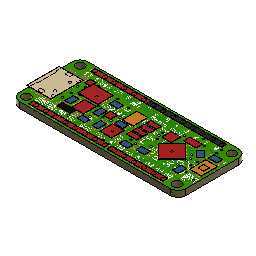
PortableEnclosure (Autodesk Fusion 360 archive; units mm, degrees)
design "Metro Mini Rev B"
part number: 20609
part number: 0.1uF
part number: YELLOW
part number: FIDUCIAL""
part number: CSTCE16M0V53-R0 16MHZ
part number: KMR2
part number: 20610
part number: MBR120
part number: 1K
part number: MIC5225-3.3
part number: ATMEGA328P
part number: CP2104
part number: 20329
Autodesk Fusion 360 part; units mm, degrees
sketch "sketch 301" plane through (0, 0, 0) normal (0, 0, 1) x (1, 0, 0)
  line L0 (0, 15.748) -> (0, 11.684)
  line L1 (0, 11.684) -> (0.254, 11.43)
  line L2 (0.254, 11.43) -> (0.254, 6.604)
  line L3 (0.254, 6.604) -> (0, 6.35)
  line L4 (0, 6.35) -> (0, 2.032)
  arc A0 (0, 2.032) -> (2.032, 0) centre (2.032, 2.032) ccw
  line L5 (2.032, 0) -> (41.148, 0)
  arc A1 (41.148, 0) -> (43.18, 2.032) centre (41.148, 2.032) ccw
  line L6 (43.18, 2.032) -> (43.18, 15.748)
  arc A2 (43.18, 15.748) -> (41.148, 17.78) centre (41.148, 15.748) ccw
  line L7 (41.148, 17.78) -> (2.032, 17.78)
  arc A3 (2.032, 17.78) -> (0, 15.748) centre (2.032, 15.748) ccw
  circle A4 centre (1.905, 15.875) radius 1.1
  circle A5 centre (1.905, 1.905) radius 1.1
  circle A6 centre (41.275, 15.875) radius 1.1
  circle A7 centre (41.021, 1.905) radius 1.1
  arc A8 (3.068, 12.59) -> (2.718, 12.94) centre (2.718, 12.59) ccw
  line L8 (3.068, 12.59) -> (3.068, 12.39)
  arc A9 (2.718, 12.04) -> (3.068, 12.39) centre (2.718, 12.39) ccw
  line L9 (2.718, 12.04) -> (2.168, 12.04)
  arc A10 (1.768, 12.39) -> (2.168, 12.04) centre (2.143, 12.415) ccw
  line L10 (1.768, 12.39) -> (1.768, 12.59)
  arc A11 (2.168, 12.94) -> (1.768, 12.59) centre (2.143, 12.565) ccw
  line L11 (2.168, 12.94) -> (2.718, 12.94)
  arc A12 (2.718, 4.84) -> (3.068, 5.29) centre (2.668, 5.24) ccw
  line L12 (2.718, 4.84) -> (2.118, 4.84)
  arc A13 (1.768, 5.29) -> (2.118, 4.84) centre (2.168, 5.24) ccw
  arc A14 (2.118, 5.74) -> (1.768, 5.29) centre (2.168, 5.34) ccw
  line L13 (2.118, 5.74) -> (2.718, 5.74)
  arc A15 (3.068, 5.29) -> (2.718, 5.74) centre (2.668, 5.34) ccw
extrude "Board" add sketch "sketch 301" along normal blind 1.57 makes body 1 in component "Board"
sketch "sketch 1110" plane through (0, 0, 0) normal (0, 0, 1) x (1, 0, 0)
  line L0 (-7.62, -0.635) -> (6.85, -0.635)
  line L1 (6.85, -0.635) -> (6.85, 0.635)
  line L2 (6.85, 0.635) -> (-7.62, 0.635)
  line L3 (-7.62, 0.635) -> (-7.62, -0.635)
extrude "1X06_ROUND" add sketch "sketch 1110" along normal blind 0.1 separate body makes body 2 in component "1X06_ROUND"
sketch "sketch 1313" plane through (0, 0, 0) normal (0, 0, 1) x (1, 0, 0)
  line L0 (-1.092, -0.724) -> (1.106, -0.724)
  line L1 (1.106, -0.724) -> (1.106, 0.726)
  line L2 (1.106, 0.726) -> (-1.092, 0.726)
  line L3 (-1.092, 0.726) -> (-1.092, -0.724)
extrude "0805-NO" add sketch "sketch 1313" along normal blind 0.1 separate body makes body 3 in component "0805-NO"
sketch "sketch 1468" plane through (0, 0, 0) normal (0, 0, 1) x (1, 0, 0)
  line L0 (-0.625, -1.3334) -> (0.625, -1.3334)
  line L1 (0.625, -1.3334) -> (0.625, 1.3334)
  line L2 (0.625, 1.3334) -> (-0.625, 1.3334)
  line L3 (-0.625, 1.3334) -> (-0.625, -1.3334)
extrude "CHIPLED_0805_NOOUTLINE" add sketch "sketch 1468" along normal blind 0.1 separate body makes body 4 in component "CHIPLED_0805_NOOUTLINE"
sketch "sketch 1607" plane through (0, 0, 0) normal (0, 0, 1) x (1, 0, 0)
  line L0 (-0.75, -0.75) -> (0.75, -0.75)
  line L1 (0.75, -0.75) -> (0.75, 0.75)
  line L2 (0.75, 0.75) -> (-0.75, 0.75)
  line L3 (-0.75, 0.75) -> (-0.75, -0.75)
extrude "FIDUCIAL_1MM" add sketch "sketch 1607" along normal blind 0.1 separate body makes body 5 in component "FIDUCIAL_1MM"
sketch "sketch 1738" plane through (0, 0, 0) normal (0, 0, 1) x (1, 0, 0)
  line L0 (-1, -0.65) -> (1, -0.65)
  line L1 (1, -0.65) -> (1, 0.65)
  line L2 (1, 0.65) -> (-1, 0.65)
  line L3 (-1, 0.65) -> (-1, -0.65)
extrude "_0805MP" add sketch "sketch 1738" along normal blind 0.1 separate body makes body 6 in component "_0805MP"
sketch "sketch 1869" plane through (0, 0, 0) normal (0, 0, 1) x (1, 0, 0)
  line L0 (-1.6, -0.8) -> (1.6, -0.8)
  line L1 (1.6, -0.8) -> (1.6, 0.8)
  line L2 (1.6, 0.8) -> (-1.6, 0.8)
  line L3 (-1.6, 0.8) -> (-1.6, -0.8)
extrude "RESONATOR" add sketch "sketch 1869" along normal blind 0.1 separate body makes body 7 in component "RESONATOR"
sketch "sketch 2000" plane through (0, 0, 0) normal (0, 0, 1) x (1, 0, 0)
  line L0 (-2.1, -1.525) -> (2.1, -1.525)
  line L1 (2.1, -1.525) -> (2.1, 1.525)
  line L2 (2.1, 1.525) -> (-2.1, 1.525)
  line L3 (-2.1, 1.525) -> (-2.1, -1.525)
extrude "BTN_KMR2_4.6X2.8" add sketch "sketch 2000" along normal blind 0.1 separate body makes body 8 in component "BTN_KMR2_4.6X2.8"
sketch "sketch 2131" plane through (0, 0, 0) normal (0, 0, 1) x (1, 0, 0)
  line L0 (-10.16, -0.635) -> (9.39, -0.635)
  line L1 (9.39, -0.635) -> (9.39, 0.635)
  line L2 (9.39, 0.635) -> (-10.16, 0.635)
  line L3 (-10.16, 0.635) -> (-10.16, -0.635)
extrude "1X08_ROUND" add sketch "sketch 2131" along normal blind 0.1 separate body makes body 9 in component "1X08_ROUND"
sketch "sketch 2262" plane through (0, 0, 0) normal (0, 0, 1) x (1, 0, 0)
  line L0 (-2.286, -1.016) -> (2.286, -1.016)
  line L1 (2.286, -1.016) -> (2.286, 1.016)
  line L2 (2.286, 1.016) -> (-2.286, 1.016)
  line L3 (-2.286, 1.016) -> (-2.286, -1.016)
extrude "SOLDERJUMPER_2WAY_OPEN_NOPASTE" add sketch "sketch 2262" along normal blind 0.1 separate body makes body 10 in component "SOLDERJUMPER_2WAY_OPEN_NOPASTE"
sketch "sketch 2393" plane through (0, 0, 0) normal (0, 0, 1) x (1, 0, 0)
  line L0 (-1.723, -0.7) -> (1.723, -0.7)
  line L1 (1.723, -0.7) -> (1.723, 0.7)
  line L2 (1.723, 0.7) -> (-1.723, 0.7)
  line L3 (-1.723, 0.7) -> (-1.723, -0.7)
extrude "SOD-123" add sketch "sketch 2393" along normal blind 0.1 separate body makes body 11 in component "SOD-123"
sketch "sketch 2524" plane through (0, 0, 0) normal (0, 0, 1) x (1, 0, 0)
  line L0 (-1.9, -1.4) -> (1.9, -1.4)
  line L1 (1.9, -1.4) -> (1.9, 1.4)
  line L2 (1.9, 1.4) -> (-1.9, 1.4)
  line L3 (-1.9, 1.4) -> (-1.9, -1.4)
extrude "RESPACK_4X0603" add sketch "sketch 2524" along normal blind 0.1 separate body makes body 12 in component "RESPACK_4X0603"
sketch "sketch 2663" plane through (0, 0, 0) normal (0, 0, 1) x (1, 0, 0)
  line L0 (-1.65, -1.5) -> (1.65, -1.5)
  line L1 (1.65, -1.5) -> (1.65, 1.5)
  line L2 (1.65, 1.5) -> (-1.65, 1.5)
  line L3 (-1.65, 1.5) -> (-1.65, -1.5)
extrude "SOT23-5" add sketch "sketch 2663" along normal blind 0.1 separate body makes body 13 in component "SOT23-5"
sketch "sketch 2794" plane through (0, 0, 0) normal (0, 0, 1) x (1, 0, 0)
  line L0 (-2.5, -2.5) -> (2.5, -2.5)
  line L1 (2.5, -2.5) -> (2.5, 2.5)
  line L2 (2.5, 2.5) -> (-2.5, 2.5)
  line L3 (-2.5, 2.5) -> (-2.5, -2.5)
extrude "MLF32-TH" add sketch "sketch 2794" along normal blind 0.1 separate body makes body 14 in component "MLF32-TH"
sketch "sketch 2925" plane through (0, 0, 0) normal (0, 0, 1) x (1, 0, 0)
  line L0 (-10.16, -0.635) -> (9.39, -0.635)
  line L1 (9.39, -0.635) -> (9.39, 0.635)
  line L2 (9.39, 0.635) -> (-10.16, 0.635)
  line L3 (-10.16, 0.635) -> (-10.16, -0.635)
extrude "1X08_ROUND_70" add sketch "sketch 2925" along normal blind 0.1 separate body makes body 15 in component "1X08_ROUND_70"
sketch "sketch 3056" plane through (0, 0, 0) normal (0, 0, 1) x (1, 0, 0)
  line L0 (-0.002, -0.002) -> (2.436, -0.002)
  line L1 (2.436, -0.002) -> (2.436, 2.433)
  line L2 (2.436, 2.433) -> (-0.002, 2.433)
  line L3 (-0.002, 2.433) -> (-0.002, -0.002)
extrude "ADAFRUIT_2.5MM" add sketch "sketch 3056" along normal blind 0.1 separate body makes body 16 in component "ADAFRUIT_2.5MM"
sketch "sketch 3187" plane through (0, 0, 0) normal (0, 0, 1) x (1, 0, 0)
  line L0 (0.013, 0.013) -> (25.336, 0.013)
  line L1 (25.336, 0.013) -> (25.336, 12.764)
  line L2 (25.336, 12.764) -> (0.013, 12.764)
  line L3 (0.013, 12.764) -> (0.013, 0.013)
extrude "METROMINI_SILK" add sketch "sketch 3187" along normal blind 0.1 separate body makes body 17 in component "METROMINI_SILK"
sketch "sketch 3318" plane through (0, 0, 0) normal (0, 0, 1) x (1, 0, 0)
  line L0 (-0.004, -0.004) -> (4.873, -0.004)
  line L1 (4.873, -0.004) -> (4.873, 4.865)
  line L2 (4.873, 4.865) -> (-0.004, 4.865)
  line L3 (-0.004, 4.865) -> (-0.004, -0.004)
extrude "ADAFRUIT_5MM" add sketch "sketch 3318" along normal blind 0.1 separate body makes body 18 in component "ADAFRUIT_5MM"
sketch "sketch 3449" plane through (0, 0, 0) normal (0, 0, 1) x (1, 0, 0)
  line L0 (-0.006, -0.006) -> (4.032, -0.006)
  line L1 (4.032, -0.006) -> (4.032, 2.877)
  line L2 (4.032, 2.877) -> (-0.006, 2.877)
  line L3 (-0.006, 2.877) -> (-0.006, -0.006)
extrude "SYMBOL_CE_TINY" add sketch "sketch 3449" along normal blind 0.1 separate body makes body 19 in component "SYMBOL_CE_TINY"
sketch "sketch 3580" plane through (0, 0, 0) normal (0, 0, 1) x (1, 0, 0)
  line L0 (-0.006, -0.006) -> (3.981, -0.006)
  line L1 (3.981, -0.006) -> (3.981, 2.838)
  line L2 (3.981, 2.838) -> (-0.006, 2.838)
  line L3 (-0.006, 2.838) -> (-0.006, -0.006)
extrude "SYMBOL_FCC_TINY" add sketch "sketch 3580" along normal blind 0.1 separate body makes body 20 in component "SYMBOL_FCC_TINY"
sketch "sketch 3711" plane through (0, 0, 0) normal (0, 0, 1) x (1, 0, 0)
  line L0 (-3.175, -2) -> (2, -2)
  line L1 (2, -2) -> (2, 2)
  line L2 (2, 2) -> (-3.175, 2)
  line L3 (-3.175, 2) -> (-3.175, -2)
extrude "QFN24_4MM_SMSC" add sketch "sketch 3711" along normal blind 0.1 separate body makes body 21 in component "QFN24_4MM_SMSC"
sketch "sketch 3842" plane through (0, 0, 0) normal (0, 0, 1) x (1, 0, 0)
  line L0 (-4.05, -4.9) -> (4.35, -4.9)
  line L1 (4.35, -4.9) -> (4.35, 1.3)
  line L2 (4.35, 1.3) -> (-4.05, 1.3)
  line L3 (-4.05, 1.3) -> (-4.05, -4.9)
extrude "4UCONN_20329_V2" add sketch "sketch 3842" along normal blind 0.1 separate body makes body 22 in component "4UCONN_20329_V2"
sketch "sketch 3973" plane through (0, 0, 0) normal (0, 0, 1) x (1, 0, 0)
  line L0 (-0.898, -0.898) -> (0.898, -0.898)
  line L1 (0.898, -0.898) -> (0.898, 0.898)
  line L2 (0.898, 0.898) -> (-0.898, 0.898)
  line L3 (-0.898, 0.898) -> (-0.898, -0.898)
extrude "PCBFEAT-REV-040" add sketch "sketch 3973" along normal blind 0.1 separate body makes body 23 in component "PCBFEAT-REV-040"
sketch "sketch 559" plane through (0, 0, 0) normal (0, 0, 1) x (1, 0, 0)
  circle A0 centre (25.146, 5.842) radius 0.2415
  circle A1 centre (14.605, 5.715) radius 0.2415
  circle A2 centre (33.02, 8.509) radius 0.25
  circle A3 centre (39.116, 15.24) radius 0.2415
  circle A4 centre (9.271, 4.318) radius 0.2415
  circle A5 centre (21.59, 2.286) radius 0.2415
  circle A6 centre (34.29, 15.367) radius 0.2415
  circle A7 centre (38.735, 9.525) radius 0.2415
  circle A8 centre (20.701, 5.461) radius 0.2415
  circle A9 centre (26.543, 5.588) radius 0.2415
  circle A10 centre (18.669, 9.398) radius 0.2415
  circle A11 centre (10.922, 11.176) radius 0.2415
  circle A12 centre (36.068, 13.97) radius 0.2415
  circle A13 centre (11.557, 3.175) radius 0.2415
  circle A14 centre (42.291, 4.826) radius 0.2415
  circle A15 centre (28.321, 9.398) radius 0.2415
  circle A16 centre (27.686, 11.557) radius 0.2415
  circle A17 centre (16.383, 7.239) radius 0.2415
  circle A18 centre (8.763, 13.716) radius 0.25
  circle A19 centre (36.957, 8.382) radius 0.197
  circle A20 centre (36.703, 6.35) radius 0.197
  circle A21 centre (37.084, 9.398) radius 0.197
  circle A22 centre (36.322, 10.414) radius 0.197
  circle A23 centre (31.115, 13.716) radius 0.2415
  circle A24 centre (8.382, 9.398) radius 0.25
  circle A25 centre (13.335, 9.271) radius 0.25
  circle A26 centre (39.497, 5.715) radius 0.197
  circle A27 centre (17.653, 12.7) radius 0.2415
  circle A28 centre (38.608, 7.874) radius 0.197
  circle A29 centre (14.224, 13.335) radius 0.2415
  circle A30 centre (6.223, 10.922) radius 0.2415
  circle A31 centre (6.731, 6.477) radius 0.2415
  circle A32 centre (29.21, 6.985) radius 0.2415
  circle A33 centre (18.161, 7.62) radius 0.2415
  circle A34 centre (39.243, 13.97) radius 0.2415
  circle A35 centre (27.813, 10.414) radius 0.2415
  circle A36 centre (6.858, 8.636) radius 0.25
  circle A37 centre (7.366, 11.811) radius 0.25
  circle A38 centre (25.4, 1.27) radius 0.5
  circle A39 centre (27.94, 1.27) radius 0.5
  circle A40 centre (30.48, 1.27) radius 0.5
  circle A41 centre (33.02, 1.27) radius 0.5
  circle A42 centre (35.56, 1.27) radius 0.5
  circle A43 centre (38.1, 1.27) radius 0.5
  circle A44 centre (17.78, 16.51) radius 0.5
  circle A45 centre (15.24, 16.51) radius 0.5
  circle A46 centre (12.7, 16.51) radius 0.5
  circle A47 centre (10.16, 16.51) radius 0.5
  circle A48 centre (7.62, 16.51) radius 0.5
  circle A49 centre (5.08, 16.51) radius 0.5
  circle A50 centre (20.32, 16.51) radius 0.5
  circle A51 centre (22.86, 16.51) radius 0.5
  circle A52 centre (25.4, 16.51) radius 0.5
  circle A53 centre (27.94, 16.51) radius 0.5
  circle A54 centre (30.48, 16.51) radius 0.5
  circle A55 centre (33.02, 16.51) radius 0.5
  circle A56 centre (35.56, 16.51) radius 0.5
  circle A57 centre (38.1, 16.51) radius 0.5
  circle A58 centre (5.08, 1.27) radius 0.5
  circle A59 centre (7.62, 1.27) radius 0.5
  circle A60 centre (10.16, 1.27) radius 0.5
  circle A61 centre (12.7, 1.27) radius 0.5
  circle A62 centre (15.24, 1.27) radius 0.5
  circle A63 centre (17.78, 1.27) radius 0.5
  circle A64 centre (20.32, 1.27) radius 0.5
  circle A65 centre (22.86, 1.27) radius 0.5
  circle A66 centre (4.318, 10.84) radius 0.35
  circle A67 centre (4.318, 6.94) radius 0.35
  circle A68 centre (2.418, 5.29) radius 0.45
  circle A69 centre (2.418, 12.49) radius 0.45
  circle A70 centre (5.218, 12.19) radius 0.4
  circle A71 centre (5.218, 5.59) radius 0.4
extrude "Extrude2" cut sketch "sketch 559" along normal blind 1.57 bodies 1 in component "Board"
component "PCB Component" placed x (1, 0, 0) y (0, 1, 0) z (0, 0, 1) at (0, 0, 0)
component "Board" placed x (1, 0, 0) y (0, 1, 0) z (0, 0, 1) at (0, 0, 0) in component "PCB Component"
component "1X06_ROUND" placed x (1, 0, 0) y (0, 1, 0) z (0, 0, 1) at (31.75, 1.27, 1.57) in component "PCB Component"
component "1X06_ROUND" placed x (-1, 0, 0) y (0, -1, 0) z (0, 0, 1) at (11.43, 16.51, 1.57) in component "PCB Component"
component "0805-NO" placed x (0, -1, 0) y (1, 0, 0) z (0, 0, 1) at (17.653, 5.08, 1.57) in component "PCB Component"
component "0805-NO" placed x (1, 0, 0) y (0, 1, 0) z (0, 0, 1) at (29.148, 4.931, 1.57) in component "PCB Component"
component "0805-NO" placed x (-1, 0, 0) y (0, -1, 0) z (0, 0, 1) at (20.447, 8.001, 1.57) in component "PCB Component"
component "0805-NO" placed x (0, 1, 0) y (-1, 0, 0) z (0, 0, 1) at (8.509, 7.112, 1.57) in component "PCB Component"
component "0805-NO" placed x (-0.707107, 0.707107, 0) y (-0.707107, -0.707107, 0) z (0, 0, 1) at (37.27, 11.603, 1.57) in component "PCB Component"
component "0805-NO" placed x (1, 0, 0) y (0, 1, 0) z (0, 0, 1) at (25.527, 4.191, 1.57) in component "PCB Component"
component "0805-NO" placed x (1, 0, 0) y (0, 1, 0) z (0, 0, 1) at (40.386, 12.446, 1.57) in component "PCB Component"
component "0805-NO" placed x (0, -1, 0) y (1, 0, 0) z (0, 0, 1) at (38.1, 5.461, 1.57) in component "PCB Component"
component "0805-NO" placed x (1, 0, 0) y (0, 1, 0) z (0, 0, 1) at (15.367, 11.811, 1.57) in component "PCB Component"
component "0805-NO" placed x (0, -1, 0) y (1, 0, 0) z (0, 0, 1) at (14.859, 8.001, 1.57) in component "PCB Component"
component "CHIPLED_0805_NOOUTLINE" placed x (0, 1, 0) y (-1, 0, 0) z (0, 0, 1) at (24.638, 8.763, 1.57) in component "PCB Component"
component "CHIPLED_0805_NOOUTLINE" placed x (0, 1, 0) y (-1, 0, 0) z (0, 0, 1) at (24.638, 7.112, 1.57) in component "PCB Component"
component "CHIPLED_0805_NOOUTLINE" placed x (0, 1, 0) y (-1, 0, 0) z (0, 0, 1) at (24.765, 10.414, 1.57) in component "PCB Component"
component "CHIPLED_0805_NOOUTLINE" placed x (0, 1, 0) y (-1, 0, 0) z (0, 0, 1) at (24.765, 12.065, 1.57) in component "PCB Component"
component "FIDUCIAL_1MM" placed x (1, 0, 0) y (0, 1, 0) z (0, 0, 1) at (7.112, 13.335, 1.57) in component "PCB Component"
component "FIDUCIAL_1MM" placed x (1, 0, 0) y (0, 1, 0) z (0, 0, 1) at (40.894, 8.89, 1.57) in component "PCB Component"
component "_0805MP" placed x (-1, 0, 0) y (0, -1, 0) z (0, 0, 1) at (14.351, 4.318, 1.57) in component "PCB Component"
component "RESONATOR" placed x (1, 0, 0) y (0, 1, 0) z (0, 0, 1) at (33.804, 13.208, 1.57) in component "PCB Component"
component "BTN_KMR2_4.6X2.8" placed x (0, -1, 0) y (1, 0, 0) z (0, 0, 1) at (40.894, 8.89, 1.57) in component "PCB Component"
component "1X08_ROUND" placed x (1, 0, 0) y (0, 1, 0) z (0, 0, 1) at (29.21, 16.51, 1.57) in component "PCB Component"
component "SOLDERJUMPER_2WAY_OPEN_NOPASTE" placed x (1, 0, 0) y (0, -1, 0) z (0, 0, -1) at (11.811, 5.842, 0) in component "PCB Component"
component "SOD-123" placed x (-1, 0, 0) y (0, -1, 0) z (0, 0, 1) at (9.652, 4.572, 1.57) in component "PCB Component"
component "RESPACK_4X0603" placed x (0, -1, 0) y (1, 0, 0) z (0, 0, 1) at (20.955, 11.049, 1.57) in component "PCB Component"
component "SOT23-5" placed x (0, 1, 0) y (-1, 0, 0) z (0, 0, 1) at (20.701, 5.334, 1.57) in component "PCB Component"
component "SOT23-5" placed x (0, -1, 0) y (1, 0, 0) z (0, 0, 1) at (11.684, 7.112, 1.57) in component "PCB Component"
component "MLF32-TH" placed x (-0.707107, -0.707107, 0) y (0.707107, -0.707107, 0) z (0, 0, 1) at (33.02, 8.509, 1.57) in component "PCB Component"
component "1X08_ROUND_70" placed x (1, 0, 0) y (0, 1, 0) z (0, 0, 1) at (13.97, 1.27, 1.57) in component "PCB Component"
component "ADAFRUIT_2.5MM" placed x (1, 0, 0) y (0, 1, 0) z (0, 0, 1) at (28.575, 10.414, 1.57) in component "PCB Component"
component "METROMINI_SILK" placed x (-1, 0, 0) y (0, 1, 0) z (0, 0, -1) at (42.926, 2.54, 0) in component "PCB Component"
component "ADAFRUIT_5MM" placed x (-1, 0, 0) y (0, 1, 0) z (0, 0, -1) at (42.545, 9.906, 0) in component "PCB Component"
component "SYMBOL_CE_TINY" placed x (-1, 0, 0) y (0, 1, 0) z (0, 0, -1) at (11.684, 9.525, 0) in component "PCB Component"
component "SYMBOL_FCC_TINY" placed x (-1, 0, 0) y (0, 1, 0) z (0, 0, -1) at (16.383, 9.652, 0) in component "PCB Component"
component "QFN24_4MM_SMSC" placed x (1, 0, 0) y (0, 1, 0) z (0, 0, 1) at (10.922, 11.43, 1.57) in component "PCB Component"
component "4UCONN_20329_V2" placed x (0, -1, 0) y (1, 0, 0) z (0, 0, 1) at (4.318, 8.89, 1.57) in component "PCB Component"
component "PCBFEAT-REV-040" placed x (1, 0, 0) y (0, 1, 0) z (0, 0, 1) at (17.018, 8.636, 1.57) in component "PCB Component"
named bodies: "Board", "1X06_ROUND", "0805-NO", "CHIPLED_0805_NOOUTLINE", "FIDUCIAL_1MM", "_0805MP", "RESONATOR", "BTN_KMR2_4.6X2.8", "1X08_ROUND", "SOLDERJUMPER_2WAY_OPEN_NOPASTE", "SOD-123", "RESPACK_4X0603", "SOT23-5", "MLF32-TH", "1X08_ROUND_70", "ADAFRUIT_2.5MM", "METROMINI_SILK", "ADAFRUIT_5MM", "SYMBOL_CE_TINY", "SYMBOL_FCC_TINY", "QFN24_4MM_SMSC", "4UCONN_20329_V2", "PCBFEAT-REV-040"

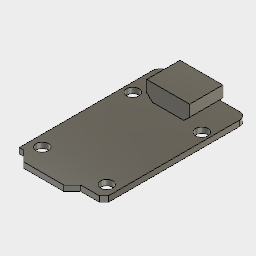
design "1501 Trinket 5V"
Autodesk Fusion 360 part; units mm, degrees
sketch "remake" plane through (0, 0, 0) normal (0, 0, 1) x (1, 0, 0)
  line L0 (-7.62, -13.32) -> (7.62, -13.32)
  line L1 (7.62, -13.32) -> (7.62, 13.32)
  line L2 (7.62, 13.32) -> (-7.62, 13.32)
  line L3 (-7.62, 13.32) -> (-7.62, -13.32)
  line L4 (-7.62, -13.32) -> (7.62, 13.32) construction
  line L5 (7.62, -13.32) -> (-7.62, 13.32) construction
  circle A0 centre (-6.1, 6.3) radius 1.1
  line L6 (0, 13.32) -> (0, 0) construction
  circle A1 centre (6.1, 6.3) radius 1.1
  circle A2 centre (-5.34, -10.2) radius 1.09
  circle A3 centre (5.34, -10.2) radius 1.09
  dimension "d3" = 26.64
  dimension "d4" = 15.24
  dimension "d5" = 2.2
  dimension "d6" = 6.3
  dimension "d7" = 6.1
  dimension "d13" = 2.18
  dimension "d14" = 5.34
  dimension "d15" = 16.5
  measures "d3" distance of L0.end L1.end
  measures "d4" distance of L1.end L2.end
  measures "d5" diameter of A0
  measures "d6" distance of L6.end A0.centre
  measures "d7" distance of L6.end A0.centre
  measures "d13" diameter of A2
  measures "d14" distance of L6.end A2.centre
  measures "d15" distance of A0.centre A2.centre
extrude "Extrude2" add sketch "remake" along normal blind 1 makes body 1
sketch "remake tester" plane through (0, 0, 0) normal (0, 0, -1) x (1, 0, 0)
  circle A0 centre (-5.34, 10.2) radius 1.09
  circle A1 centre (6.1, -6.3) radius 1.1
  circle A2 centre (5.34, 10.2) radius 1.09
  circle A3 centre (-6.1, -6.3) radius 1.1
  line L0 (-7.62, 13.32) -> (-7.62, -13.32) construction
  line L1 (-7.62, -13.32) -> (7.62, -13.32) construction
  line L2 (7.62, -13.32) -> (7.62, 13.32) construction
  line L3 (7.62, 13.32) -> (-7.62, 13.32) construction
  circle A4 centre (-5.34, 10.2) radius 2.5
  circle A5 centre (5.34, 10.2) radius 2.5
  circle A6 centre (-6.1, -6.3) radius 2.5
  circle A7 centre (6.1, -6.3) radius 2.5
  line L4 (-9.62, -15.32) -> (9.62, -15.32)
  line L5 (9.62, -15.32) -> (9.62, 15.32)
  line L6 (9.62, 15.32) -> (-9.62, 15.32)
  line L7 (-9.62, 15.32) -> (-9.62, -15.32)
  dimension "d18" = 5
  dimension "d19" = 5
  dimension "d20" = 5
  dimension "d21" = 5
  dimension "d22" = 2
  measures "d18" diameter of A4
  measures "d19" diameter of A5
  measures "d20" diameter of A6
  measures "d21" diameter of A7
extrude "Extrude3" add sketch "remake tester" along normal blind 3 and the other way blind -2 separate body contours A0 | A1 | A2 | A3 | A4 | A5 | A6 | A7 | L4 L5 L6 L7 makes body 2
extrude "Extrude4" add sketch "remake tester" along normal blind 2 contours A0 | A1 | A2 | A3 | A4 | A5 | A6 | A7 bodies 2
extrude "Extrude5" add sketch "remake tester" against normal blind 2 contours A0 | A1 | A2 | A3 bodies 2
sketch "trinket import" plane through (0, 0, 0) normal (0, 0, 1) x (1, 0, 0)
  line L0 (2.7, 13.8) -> (2.5, 13.5)
  line L1 (2.5, 13.5) -> (-2.6, 13.5)
  line L2 (-2.6, 13.5) -> (-2.8, 13.8)
  line L3 (-2.8, 13.8) -> (-6.4, 13.8)
  spline S0 degree 3 poles (-6.4, 13.8) (-7.1, 13.8) (-7.7, 13.2) (-7.7, 12.5) knots 0 0 0 0 1 1 1 1
  line L4 (-7.7, 12.5) -> (-7.7, -11.1)
  line L5 (-7.7, -11.1) -> (-6.9, -11.1)
  line L6 (-6.9, -11.1) -> (-5.1, -12.9)
  line L7 (-5.1, -12.9) -> (2, -12.9)
  line L8 (2, -12.9) -> (3.5, -11.4)
  line L9 (3.5, -11.4) -> (6.8, -11.4)
  line L10 (6.8, -11.4) -> (7.6, -10.6)
  line L11 (7.6, -10.6) -> (7.6, 12.6)
  spline S1 degree 3 poles (7.6, 12.6) (7.6, 13.3) (7, 13.9) (6.3, 13.9) knots 0 0 0 0 1 1 1 1
  line L12 (6.3, 13.9) -> (2.7, 13.9)
  line L13 (2.7, 13.9) -> (2.7, 13.8)
  circle A0 centre (-6.1, 7.4) radius 1.105
  circle A1 centre (6.1, 7.4) radius 1.105
  circle A2 centre (-5.7, -9) radius 1.09
  circle A3 centre (5.7, -9) radius 1.09
  dimension "d30" = 2.21
  dimension "d31" = 2.21
  dimension "d32" = 2.18
  dimension "d33" = 2.18
  measures "d30" diameter of A0
  measures "d31" diameter of A1
  measures "d32" diameter of A2
  measures "d33" diameter of A3
extrude "Extrude6" add sketch "trinket import" along normal blind 1 separate body makes body 3
sketch "trinket tester" plane through (0, 0, 0) normal (0, 0, -1) x (1, 0, 0)
  circle A0 centre (-6.1, -7.4) radius 1.105
  circle A1 centre (5.7, 9) radius 1.09
  circle A2 centre (6.1, -7.4) radius 1.105
  circle A3 centre (-5.7, 9) radius 1.09
  line L0 (2.7, -13.8) -> (2.7, -13.9)
  line L1 (2.7, -13.9) -> (6.3, -13.9)
  spline S0 degree 3 poles (7.6, -12.6) (7.6, -13.3) (7, -13.9) (6.3, -13.9) knots 0 0 0 0 1 1 1 1
  line L2 (7.6, -12.6) -> (7.6, 10.6) construction
  line L3 (7.6, 10.6) -> (6.8, 11.4)
  line L4 (6.8, 11.4) -> (3.5, 11.4) construction
  line L5 (3.5, 11.4) -> (2, 12.9)
  line L6 (2, 12.9) -> (-5.1, 12.9)
  line L7 (-5.1, 12.9) -> (-6.9, 11.1) construction
  line L8 (-6.9, 11.1) -> (-7.7, 11.1) construction
  line L9 (-7.7, 11.1) -> (-7.7, -12.5) construction
  spline S1 degree 3 poles (-6.4, -13.8) (-7.1, -13.8) (-7.7, -13.2) (-7.7, -12.5) knots 0 0 0 0 1 1 1 1
  line L10 (-6.4, -13.8) -> (-2.8, -13.8)
  line L11 (-2.8, -13.8) -> (-2.6, -13.5)
  line L12 (-2.6, -13.5) -> (2.5, -13.5)
  line L13 (2.5, -13.5) -> (2.7, -13.8)
  circle A4 centre (-5.7, 9) radius 3
  circle A5 centre (5.7, 9) radius 3
  circle A6 centre (-6.1, -7.4) radius 3
  circle A7 centre (6.1, -7.4) radius 3
  line L14 (-10, -13.5) -> (10, -13.5)
  line L15 (10, -13.5) -> (10, 13.5)
  line L16 (10, 13.5) -> (-10, 13.5)
  line L17 (-10, 13.5) -> (-10, -13.5)
  line L18 (-10, -13.5) -> (10, 13.5) construction
  line L19 (10, -13.5) -> (-10, 13.5) construction
  dimension "d36" = 6
  dimension "d37" = 6
  dimension "d38" = 6
  dimension "d39" = 6
  dimension "d40" = 20
  dimension "d41" = 27
  measures "d36" diameter of A4
  measures "d37" diameter of A5
  measures "d38" diameter of A6
  measures "d39" diameter of A7
  measures "d40" distance of L15.end L16.end
  measures "d41" distance of L14.end L15.end
extrude "Extrude7" add sketch "trinket tester" along normal blind 4 and the other way blind -3 separate body contours A0 | A1 | A2 | A3 | L12 L14 L15 L16 L17 | A4 | A5 | A6 | A7 makes body 4
extrude "Extrude8" add sketch "trinket tester" along normal up to surface (3 mm away) contours A0 | A1 | A2 | A3 | A4 | A5 | A6 | A7 bodies 4
extrude "Extrude9" cut sketch "trinket tester" along normal blind 10 contours A0 | A1 | A2 | A3 bodies 4
chamfer "Chamfer1" distance 1 angle 45 4 edges at (-6.7162, -9.3942, -4) (4.6838, -9.3942, -4) (-7.1302, 7.0004, -4) (5.0698, 7.0004, -4) on bodies 4
sketch "Sketch12" plane through (0, 13.5, 0) normal (0, 1, 0) x (-1, 0, 0)
  line L0 (-2.5, 0) -> (2.6, 0)
  line L1 (2.6, 0) -> (2.6, 1)
  line L2 (2.6, 1) -> (-2.5, 1)
  line L3 (-2.5, 1) -> (-2.5, 0)
  line L4 (0.05, 1) -> (0.05, 3.5) construction
  line L5 (3.85, 1) -> (-3.75, 1)
  line L6 (-3.75, 1) -> (-3.75, 4)
  line L7 (-3.75, 4) -> (3.85, 4)
  line L8 (3.85, 4) -> (3.85, 1)
  line L9 (3.85, 1) -> (-3.75, 4) construction
  line L10 (-3.75, 1) -> (3.85, 4) construction
  point P0 (0.05, 2.5)
  dimension "d49" = 7.6
  dimension "d50" = 3
  measures "d49" distance of L6.end L7.end
  measures "d50" distance of L5.end L6.end
extrude "Extrude10" add sketch "Sketch12" against normal blind 5.9 separate body contours L2 L5 L6 L7 L8 makes body 5
chamfer "Chamfer2" distance 1 angle 45 2 edges at (3.75, 10.55, 1) (-3.85, 10.55, 1) on bodies 5
hidden bodies 1 2 4
named bodies: "trinket PCB", "trinket tester", "MicroUSB"

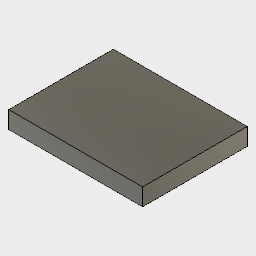
design "328 2500mAh battery"
Autodesk Fusion 360 part; units mm, degrees
sketch "Sketch1" plane through (0, 0, 0) normal (0, 0, 1) x (1, 0, 0)
  line L0 (0, 0) -> (61, 0)
  line L1 (61, 0) -> (61, -47.7)
  line L2 (61, -47.7) -> (0, -47.7)
  line L3 (0, -47.7) -> (0, 0)
  dimension "d1" = 61
  dimension "d2" = 47.7
  measures "d1" distance of L0.start L0.end
  measures "d2" distance of L0.start L2.end
extrude "Extrude1" add sketch "Sketch1" along normal blind 7.9
